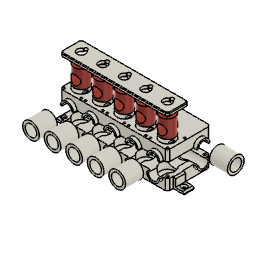
Luftstromverteilerkasten (Autodesk Fusion 360 design; units mm, degrees)
Autodesk Fusion 360 part; units mm, degrees
sketch "Skizze1" plane through (0, 0, 0) normal (0, 0, 1) x (1, 0, 0)
  line L0 (7, 22) -> (-8, 22)
  line L1 (-8, 22) -> (-8, -8)
  line L2 (-8, -8) -> (7, -8)
  line L3 (7, 22) -> (22, 22)
  line L4 (22, 22) -> (22, -8)
  line L5 (22, -8) -> (7, -8)
  line L6 (0.25, -0.3782) -> (0.25, -8)
  line L7 (0.25, -8) -> (7, -8)
  line L8 (13.75, -0.3782) -> (13.75, -8)
  line L9 (13.75, -8) -> (7, -8)
  circle A0 centre (7, 7) radius 10
  line L10 (0.25, -8) -> (0.25, 22)
  line L11 (13.75, -8) -> (13.75, 22)
  circle A1 centre (7, 7) radius 10.25
  dimension "d6" = 15
  dimension "d7" = 30
  dimension "d8" = 15
  dimension "d9" = 30
  dimension "d14" = 20
  dimension "d15" = 20.5
  constraint horizontal L0
  constraint vertical L1
  constraint horizontal L2
  constraint horizontal L3
  constraint vertical L4
  constraint horizontal L5
  constraint vertical L6
  constraint horizontal L7
  constraint vertical L8
  constraint horizontal L9
  constraint coincident A0 L6.start
  constraint coincident A0 L8.start
  constraint coincident L0 L10.end
  constraint perpendicular L0 L10
  constraint coincident L3 L11.end
  constraint perpendicular L3 L11
  constraint concentric A0 A1
  measures "d6" distance of L0.start L0.end
  measures "d7" distance of L0.start L2.end
  measures "d8" distance of L0.start L3.end
  measures "d9" distance of L0.start L2.end
  measures "d14" diameter of A0
  measures "d15" diameter of A1
  measures "d43" distance of L2.end
  measures "d44" distance of L2.end
extrude "Extrusion1" add sketch "Skizze1" along normal blind 30 contours L0 L3 L10 L11 A1 | L0 L1 L2 L6 L10 A1 | L3 L4 L5 L8 L11 A1 | L2 L5 L6 L7 L8 L9 L10 L11 A1 makes body 1
sketch "Skizze2" plane through (0, -8, 0) normal (0, -1, 0) x (1, 0, 0)
  line L0 (-8, 0) -> (22, 0)
  line L1 (22, 0) -> (22, 30)
  line L2 (22, 30) -> (-8, 30)
  line L3 (-8, 30) -> (-8, 0)
  line L4 (-8, 30) -> (22, 0)
  circle A0 centre (7, 15) radius 6.75
  dimension "d18" = 13.5
  constraint coincident L2.end L3.start
  constraint coincident L0.end L1.start
  constraint midpoint L4 A0.centre
  measures "d18" diameter of A0
extrude "Extrusion2" cut sketch "Skizze2" against normal blind 50 contours L4 A0 | L4 A0 bodies 1
extrude "Extrusion3" add sketch "Skizze1" along normal blind 5 contours A0 L10 L11 A1 | L6 A0 L10 A1 | L8 A0 L11 A1 | A0 L10 | A0 L10 L11 | L6 L8 A0 L10 L11 A1 | A0 L11 bodies 1
sketch "Skizze3" plane through (0, 0, 0) normal (0, 0, -1) x (1, 0, 0)
  line L0 (-8, -22) -> (22, -22)
  line L1 (22, -22) -> (22, 8)
  line L2 (22, 8) -> (-8, 8)
  line L3 (-8, 8) -> (-8, -22)
sketch "Skizze4" plane through (0, 0, 5) normal (0, 0, 1) x (-1, 0, 0)
  circle A0 centre (-7, -7) radius 10.25
  circle A1 centre (-7, -7) radius 2
  constraint concentric A0 A1
extrude "Extrusion4" add sketch "Skizze4" along normal blind 1 contours A1 bodies 1
sketch "Skizze5" plane through (0, 0, 5) normal (0, 0, 1) x (-1, 0, 0)
  circle A0 centre (-7, -7) radius 2
  circle A1 centre (-7, -7) radius 10.25
  circle A2 centre (-7, -7) radius 10
  circle A3 centre (-7, -7) radius 2.5
  dimension "d25" = 5
  constraint concentric A0 A2
  constraint concentric A2 A3
  measures "d25" diameter of A3
extrude "Extrusion5" add sketch "Skizze5" along normal blind 24.7 separate body contours A2 makes body 2
move_body "Verschieben1" bodies 2 to x (1, 0, 0) y (0, 1, 0) z (0, 0, 1) at (0, 0, 57)
sketch "Skizze6" plane through (0, 0, 86.7) normal (0, 0, 1) x (-1, 0, 0)
  circle A0 centre (-7, -7) radius 2.5
  circle A1 centre (-7, -7) radius 10
  circle A2 centre (-7, -7) radius 10
  constraint concentric A0 A2
extrude "Extrusion6" add sketch "Skizze6" against normal blind 23 contours A0 bodies 2
extrude "Extrusion7" add 1 faces at (8.044, 7.2271, 63.7) along direction (0, 0, -1) blind 0.7 on bodies 2 bodies 2
move_body "Verschieben2" bodies 2 to x (1, 0, 0) y (0, 1, 0) z (0, 0, 1) at (0, 0, -56.7)
extrude "Extrusion8" cut sketch "Skizze2" against normal blind 133 contours L4 A0 | L4 A0 bodies 2
sketch "Skizze7" plane through (0, 0, 30) normal (0, 0, 1) x (-1, 0, 0)
  circle A0 centre (-7, -7) radius 10
  circle A1 centre (-7, -7) radius 2.35
  dimension "d34" = 4.7
  constraint concentric A0 A1
  measures "d34" diameter of A1
extrude "Extrusion9" cut sketch "Skizze7" against normal blind 3.2 contours A1 bodies 2
sketch "Skizze8" plane through (0, 0, 30) normal (0, 0, 1) x (-1, 0, 0)
  circle A0 centre (-7, -7) radius 10.25
  line L0 (-22, -22) -> (8, -22)
  line L1 (8, -22) -> (8, 8)
  line L2 (8, 8) -> (-22, 8)
  line L3 (-22, 8) -> (-22, -22)
  line L4 (-22, -22) -> (8, 8)
  line L5 (8, -22) -> (-22, 8)
  line L6 (8, -22) -> (5, -22)
  line L7 (5, -22) -> (5, -19)
  line L8 (5, -19) -> (8, -19)
  line L9 (8, -19) -> (8, -22)
  line L10 (-22, -22) -> (-19, -22)
  line L11 (-19, -22) -> (-19, -19)
  line L12 (-19, -19) -> (-22, -19)
  line L13 (-22, -19) -> (-22, -22)
  line L14 (8, 8) -> (5, 8)
  line L15 (5, 8) -> (5, 5)
  line L16 (5, 5) -> (8, 5)
  line L17 (8, 5) -> (8, 8)
  line L18 (-22, 8) -> (-19, 8)
  line L19 (-19, 8) -> (-19, 5)
  line L20 (-19, 5) -> (-22, 5)
  line L21 (-22, 5) -> (-22, 8)
  circle A1 centre (5, 5) radius 1.5
  circle A2 centre (-19, 5) radius 1.5
  circle A3 centre (-19, -19) radius 1.5
  circle A4 centre (5, -19) radius 1.5
  dimension "d37" = 3
  dimension "d38" = 3
  dimension "d39" = 3
  dimension "d40" = 3
  dimension "d41" = 3
  dimension "d42" = 3
  dimension "d43" = 3
  dimension "d44" = 3
  constraint coincident L0.start L3.end
  constraint coincident L1.end L2.start
  constraint coincident L0.end L1.start
  constraint coincident L2.end L3.start
  constraint horizontal L6
  constraint vertical L7
  constraint horizontal L8
  constraint vertical L9
  constraint horizontal L10
  constraint vertical L11
  constraint horizontal L12
  constraint vertical L13
  constraint horizontal L14
  constraint vertical L15
  constraint horizontal L16
  constraint vertical L17
  constraint horizontal L18
  constraint vertical L19
  constraint horizontal L20
  constraint vertical L21
  constraint coincident L15.end L16.start
  constraint coincident L19.end L20.start
  constraint coincident L11.end L12.start
  constraint coincident L7.end L8.start
  measures "d37" distance of L0.end L6.end
  measures "d38" distance of L0.end L8.end
  measures "d39" distance of L0.start L10.end
  measures "d40" distance of L0.start L12.end
  measures "d41" distance of L1.end L14.end
  measures "d42" distance of L1.end L16.end
  measures "d43" distance of L2.end L18.end
  measures "d44" distance of L2.end L20.end
extrude "Extrusion10" cut sketch "Skizze8" against normal blind 2 contours L4 L15 A1 | L4 L16 A1 | L5 L8 A4 | L5 L7 A4 | L5 L20 A2 | L5 L19 A2 | L4 L15 A1 | L4 L16 A1 | L4 L11 A3 | L4 L12 A3 | L5 L8 A4 | L5 L7 A4 | L5 L20 A2 | L5 L19 A2 | L4 L11 A3 | L4 L12 A3 bodies 1
copy_body "Körper kopieren/einfügen1" bodies 2 1 makes body 3 makes body 4
move_body "Verschieben3" bodies 3 4 to x (1, 0, 0) y (0, 1, 0) z (0, 0, 1) at (30, 0, 0)
copy_body "Körper kopieren/einfügen2" bodies 3 4 1 2 makes body 5 makes body 6 makes body 7 makes body 8
move_body "Verschieben4" bodies 5 6 7 8 to x (1, 0, 0) y (0, 1, 0) z (0, 0, 1) at (60, 0, 0)
copy_body "Körper kopieren/einfügen3" bodies 5 6 makes body 9 makes body 10
move_body "Verschieben5" bodies 9 10 to x (1, 0, 0) y (0, 1, 0) z (0, 0, 1) at (30, 0, 0)
combine "Kombinieren1" operation add target body 1 tool bodies 4 7 6 10
sketch "Skizze9" plane through (0, 0, 0) normal (0, 1, 0) x (1, 0, 0)
sketch "Skizze10" plane through (0, 0, 30) normal (0, 0, 1) x (-1, 0, 0)
  circle A0 centre (-127, -7) radius 10.25
  circle A1 centre (-115, 5) radius 1.5
  circle A2 centre (-115, -19) radius 1.5
  circle A3 centre (-139, 5) radius 1.5
  circle A4 centre (-139, -19) radius 1.5
  circle A5 centre (-97, -7) radius 10.25
  circle A6 centre (-85, 5) radius 1.5
  circle A7 centre (-85, -19) radius 1.5
  circle A8 centre (-109, 5) radius 1.5
  circle A9 centre (-109, -19) radius 1.5
  circle A10 centre (-67, -7) radius 10.25
  circle A11 centre (-55, 5) radius 1.5
  circle A12 centre (-55, -19) radius 1.5
  circle A13 centre (-79, 5) radius 1.5
  circle A14 centre (-79, -19) radius 1.5
  circle A15 centre (-37, -7) radius 10.25
  circle A16 centre (-25, 5) radius 1.5
  circle A17 centre (-25, -19) radius 1.5
  circle A18 centre (-49, 5) radius 1.5
  circle A19 centre (-49, -19) radius 1.5
  circle A20 centre (-19, -19) radius 1.5
  circle A21 centre (-19, 5) radius 1.5
  circle A22 centre (5, -19) radius 1.5
  circle A23 centre (5, 5) radius 1.5
  circle A24 centre (-7, -7) radius 10.25
  line L0 (-142, -22) -> (8, -22)
  line L1 (8, -22) -> (8, 8)
  line L2 (8, 8) -> (-142, 8)
  line L3 (-142, 8) -> (-142, -22)
  line L4 (8, -22) -> (-142, -22)
  line L5 (-142, -22) -> (-142, 8)
  line L6 (-142, 8) -> (8, 8)
  line L7 (8, 8) -> (8, -22)
  circle A25 centre (-7, -7) radius 5.9
  circle A26 centre (-37, -7) radius 5.9
  circle A27 centre (-67, -7) radius 5.9
  circle A28 centre (-97, -7) radius 5.9
  circle A29 centre (-127, -7) radius 5.9
  line L8 (-7, -7) -> (-7, -15.8)
  line L9 (-37, -7) -> (-37, -15.8)
  line L10 (-67, -7) -> (-67, -15.8)
  line L11 (-97, -7) -> (-97, -15.8)
  line L12 (-127, -7) -> (-127, -15.8)
  circle A30 centre (-7, -13.3) radius 2.5
  circle A31 centre (-37, -13.3) radius 2.5
  circle A32 centre (-67, -13.3) radius 2.5
  circle A33 centre (-97, -13.3) radius 2.5
  circle A34 centre (-127, -13.3) radius 2.5
  line L13 (-7, -13.3) -> (-4.5, -13.3)
  line L14 (-4.5, -13.3) -> (-4.5, -12.3442)
  line L15 (-7, -13.3) -> (-9.5, -13.3)
  line L16 (-9.5, -13.3) -> (-9.5, -12.3442)
  line L17 (-37, -13.3) -> (-34.5, -13.3)
  line L18 (-34.5, -13.3) -> (-34.5, -12.3442)
  line L19 (-37, -13.3) -> (-39.5, -13.3)
  line L20 (-39.5, -13.3) -> (-39.5, -12.3442)
  line L21 (-67, -13.3) -> (-64.5, -13.3)
  line L22 (-64.5, -13.3) -> (-64.5, -12.3442)
  line L23 (-67, -13.3) -> (-69.5, -13.3)
  line L24 (-69.5, -13.3) -> (-69.5, -12.3442)
  line L25 (-97, -13.3) -> (-94.5, -13.3)
  line L26 (-94.5, -13.3) -> (-94.5, -12.3442)
  line L27 (-97, -13.3) -> (-99.5, -13.3)
  line L28 (-99.5, -13.3) -> (-99.5, -12.3442)
  line L29 (-127, -13.3) -> (-124.5, -13.3)
  line L30 (-124.5, -13.3) -> (-124.5, -12.3442)
  line L31 (-127, -13.3) -> (-129.5, -13.3)
  line L32 (-129.5, -13.3) -> (-129.5, -12.3442)
  circle A35 centre (5, -19) radius 1.3
  circle A36 centre (-19, -19) radius 1.3
  circle A37 centre (-25, -19) radius 1.3
  circle A38 centre (-49, -19) radius 1.3
  circle A39 centre (-55, -19) radius 1.3
  circle A40 centre (-79, -19) radius 1.3
  circle A41 centre (-85, -19) radius 1.3
  circle A42 centre (-109, -19) radius 1.3
  circle A43 centre (-115, -19) radius 1.3
  circle A44 centre (-139, -19) radius 1.3
  circle A45 centre (-139, 5) radius 1.3
  circle A46 centre (-115, 5) radius 1.3
  circle A47 centre (-109, 5) radius 1.3
  circle A48 centre (-85, 5) radius 1.3
  circle A49 centre (-79, 5) radius 1.3
  circle A50 centre (-55, 5) radius 1.3
  circle A51 centre (-49, 5) radius 1.3
  circle A52 centre (-25, 5) radius 1.3
  circle A53 centre (-19, 5) radius 1.3
  circle A54 centre (5, 5) radius 1.3
  dimension "d47" = 11.8
  dimension "d48" = 11.8
  dimension "d49" = 11.8
  dimension "d50" = 11.8
  dimension "d51" = 11.8
  dimension "d52" = 8.8
  dimension "d53" = 8.8
  dimension "d54" = 8.8
  dimension "d55" = 8.8
  dimension "d56" = 8.8
  dimension "d57" = 5
  dimension "d58" = 5
  dimension "d59" = 5
  dimension "d60" = 5
  dimension "d61" = 5
  dimension "d62" = 2.6
  dimension "d63" = 2.6
  dimension "d64" = 2.6
  dimension "d65" = 2.6
  dimension "d66" = 2.6
  dimension "d67" = 2.6
  dimension "d68" = 2.6
  dimension "d69" = 2.6
  dimension "d70" = 2.6
  dimension "d71" = 2.6
  dimension "d72" = 2.6
  dimension "d73" = 2.6
  dimension "d74" = 2.6
  dimension "d75" = 2.6
  dimension "d76" = 2.6
  dimension "d77" = 2.6
  dimension "d78" = 2.6
  dimension "d79" = 2.6
  dimension "d80" = 2.6
  dimension "d81" = 2.6
  constraint horizontal L4
  constraint vertical L5
  constraint horizontal L6
  constraint vertical L7
  constraint coincident L2.end L3.start
  constraint coincident L0.end L1.start
  constraint concentric A24 A25
  constraint concentric A15 A26
  constraint concentric A10 A27
  constraint concentric A5 A28
  constraint concentric A0 A29
  constraint coincident A24.centre A25.centre
  constraint perpendicular L4 L8
  constraint coincident A15.centre A26.centre
  constraint vertical L9
  constraint coincident A10.centre A27.centre
  constraint vertical L10
  constraint coincident A5.centre A28.centre
  constraint perpendicular L6 L11
  constraint coincident A0.centre A29.centre
  constraint vertical L12
  constraint coincident L8.end A30
  constraint coincident L9.end A31
  constraint coincident L10.end A32
  constraint coincident L11.end A33
  constraint coincident L12.end A34
  constraint coincident A30.centre L13.start
  constraint coincident A30 L13.end
  constraint perpendicular L8 L13
  constraint coincident A25 L14.end
  constraint tangent A30 L14
  constraint coincident A30 L15.end
  constraint perpendicular L8 L15
  constraint coincident A25 L16.end
  constraint perpendicular L15 L16
  constraint coincident A31.centre L17.start
  constraint coincident A31 L17.end
  constraint perpendicular L9 L17
  constraint coincident A26 L18.end
  constraint perpendicular L17 L18
  constraint coincident A31 L19.end
  constraint perpendicular L9 L19
  constraint coincident A26 L20.end
  constraint perpendicular L19 L20
  constraint coincident A32.centre L21.start
  constraint coincident A32 L21.end
  constraint perpendicular L10 L21
  constraint coincident A27 L22.end
  constraint perpendicular L21 L22
  constraint coincident A32 L23.end
  constraint perpendicular L10 L23
  constraint perpendicular L23 L24
  constraint coincident A33.centre L25.start
  constraint coincident A33 L25.end
  constraint perpendicular L11 L25
  constraint coincident A28 L26.end
  constraint perpendicular L25 L26
  constraint coincident A33 L27.end
  constraint perpendicular L11 L27
  constraint coincident A28 L28.end
  constraint perpendicular L27 L28
  constraint coincident A34.centre L29.start
  constraint coincident A34 L29.end
  constraint perpendicular L12 L29
  constraint coincident A29 L30.end
  constraint perpendicular L29 L30
  constraint coincident A34 L31.end
  constraint perpendicular L12 L31
  constraint coincident A29 L32.end
  constraint perpendicular L29 L32
  constraint concentric A22 A35
  constraint concentric A20 A36
  constraint concentric A17 A37
  constraint concentric A19 A38
  constraint concentric A12 A39
  constraint concentric A14 A40
  constraint concentric A7 A41
  constraint concentric A9 A42
  constraint concentric A2 A43
  constraint concentric A4 A44
  constraint concentric A3 A45
  constraint concentric A1 A46
  constraint concentric A8 A47
  constraint concentric A6 A48
  constraint concentric A13 A49
  constraint concentric A11 A50
  constraint concentric A18 A51
  constraint concentric A16 A52
  constraint concentric A21 A53
  constraint concentric A23 A54
  measures "d47" diameter of A25
  measures "d48" diameter of A26
  measures "d49" diameter of A27
  measures "d50" diameter of A28
  measures "d51" diameter of A29
  measures "d52" distance of A24.centre L8.end
  measures "d53" distance of A15.centre L9.end
  measures "d54" distance of A10.centre L10.end
  measures "d55" distance of A5.centre L11.end
  measures "d56" distance of A0.centre L12.end
  measures "d57" diameter of A30
  measures "d58" diameter of A31
  measures "d59" diameter of A32
  measures "d60" diameter of A33
  measures "d61" diameter of A34
  measures "d62" diameter of A35
  measures "d63" diameter of A36
  measures "d64" diameter of A37
  measures "d65" diameter of A38
  measures "d66" diameter of A39
  measures "d67" diameter of A40
  measures "d68" diameter of A41
  measures "d69" diameter of A42
  measures "d70" diameter of A43
  measures "d71" diameter of A44
  measures "d72" diameter of A45
  measures "d73" diameter of A46
  measures "d74" diameter of A47
  measures "d75" diameter of A48
  measures "d76" diameter of A49
  measures "d77" diameter of A50
  measures "d78" diameter of A51
  measures "d79" diameter of A52
  measures "d80" diameter of A53
  measures "d81" diameter of A54
move_body "Verschieben6" bodies 1 5 8 to x (1, 0, 0) y (0, 1, 0) z (0, 0, 1) at (0, 0, -15)
move_body "Verschieben7" bodies 2 3 9 to x (1, 0, 0) y (0, 1, 0) z (0, 0, 1) at (0, 0, -15)
extrude "Extrusion11" add sketch "Skizze10" along normal blind 2 separate body contours A0 | A1 | A2 | A3 | A4 | A5 | A6 | A7 | A8 | A9 | A10 | A11 | A12 | A13 | A14 | A15 | A16 | A17 | A18 | A19 | A20 | A21 | A22 | A23 | A24 | L0 L1 L2 L3 L4 L5 L6 L7 | A35 | A36 | A37 | A38 | A39 | A40 | A41 | A42 | A43 | A44 | A45 | A46 | A47 | A48 | A49 | A50 | A51 | A52 | A53 | A54 makes body 11
extrude "Extrusion12" add sketch "Skizze10" against normal blind 2 contours A35 | A36 | A37 | A38 | A39 | A40 | A41 | A42 | A43 | A44 | A45 | A46 | A47 | A48 | A49 | A50 | A51 | A52 | A53 | A54 bodies 11
extrude "Extrusion13" cut 20 faces at (-5.1917, -5.3235, 28) (-5.3026, 18.2291, 28) (18.5623, -4.812, 28) (19.3724, 18.5636, 28) (25.3724, 18.5636, 28) (24.5623, -4.812, 28) (48.1382, -5.0646, 28) (49.0464, 18.6612, 28) (55.0464, 18.6612, 28) (54.0847, -5.0281, 28) (84.642, -5.3733, 28) (78.642, -5.3733, 28) (78.642, 18.6267, 28) (84.642, 18.6267, 28) (108.642, -5.3733, 28) (114.642, -5.3733, 28) (108.642, 18.6267, 28) (114.642, 18.6267, 28) (138.6823, -5.4239, 28) (138.6096, 19.188, 28) along direction (0, 0, 1) blind 0.2 on bodies 11 bodies 11
move_body "Verschieben8" bodies 11 to x (1, 0, 0) y (0, 1, 0) z (0, 0, 1) at (0, 0, 30)
move_body "Verschieben9" bodies 2 3 1 5 9 8 to x (1, 0, 0) y (0, 1, 0) z (0, 0, 1) at (-67, 0, 15)
move_body "Verschieben10" bodies 11 to x (1, 0, 0) y (0, 1, 0) z (0, 0, 1) at (-67, 0, -30)
sketch "Skizze11" plane through (0, 0, 0) normal (0, 0, 1) x (1, 0, 0)
  line L0 (-107.8085, 14.3255) -> (-82.0961, 14.3255)
  line L1 (-82.0961, 14.3255) -> (-82.0961, -4.2242)
  line L2 (-82.0961, -4.2242) -> (-107.8085, -4.2242)
  line L3 (-107.8085, -4.2242) -> (-107.8085, 14.3255)
  constraint horizontal L0
  constraint vertical L1
  constraint horizontal L2
  constraint vertical L3
extrude "Extrusion14" add sketch "Skizze11" along normal blind 15 separate body makes body 12
split "Teilen1" by plane through (0, 0, 15) normal (0, 0, 1) bodies 1 makes body 13 at (14.2202, 12.5653, 30)
extrude "Extrusion15" cut 1 faces at (-99.2377, 1.959, 15) along direction (0, 0, -1) blind 35 on bodies 12 bodies 12
sketch "Skizze12" plane through (0, -8, 0) normal (0, -1, 0) x (1, 0, 0)
  line L0 (66.75, 15) -> (75, 15)
  line L1 (75, 15) -> (75, 30)
  line L2 (75, 30) -> (-75, 30)
  line L3 (-75, 30) -> (-75, 15)
  line L4 (-75, 15) -> (-66.75, 15)
  arc A0 (-53.25, 15) -> (-66.75, 15) centre (-60, 15) ccw
  line L5 (-53.25, 15) -> (-36.75, 15)
  arc A1 (-23.25, 15) -> (-36.75, 15) centre (-30, 15) ccw
  line L6 (-23.25, 15) -> (-6.75, 15)
  arc A2 (6.75, 15) -> (-6.75, 15) centre (0, 15) ccw
  line L7 (6.75, 15) -> (23.25, 15)
  arc A3 (36.75, 15) -> (23.25, 15) centre (30, 15) ccw
  line L8 (36.75, 15) -> (53.25, 15)
  arc A4 (66.75, 15) -> (53.25, 15) centre (60, 15) ccw
  circle A5 centre (-60, 15) radius 9
  circle A6 centre (-30, 15) radius 9
  circle A7 centre (0, 15) radius 9
  circle A8 centre (30, 15) radius 9
  circle A9 centre (60, 15) radius 9
  circle A10 centre (-60, 15) radius 6.75
  circle A11 centre (-30, 15) radius 6.75
  circle A12 centre (0, 15) radius 6.75
  circle A13 centre (30, 15) radius 6.75
  circle A14 centre (60, 15) radius 6.75
  dimension "d92" = 18
  dimension "d93" = 18
  dimension "d94" = 18
  dimension "d95" = 18
  dimension "d96" = 18
  constraint concentric A0 A5
  constraint concentric A1 A6
  constraint concentric A2 A7
  constraint concentric A3 A8
  constraint concentric A4 A9
  constraint concentric A5 A10
  constraint concentric A6 A11
  constraint concentric A7 A12
  constraint concentric A8 A13
  constraint concentric A9 A14
  measures "d92" diameter of A5
  measures "d93" diameter of A6
  measures "d94" diameter of A7
  measures "d95" diameter of A8
  measures "d96" diameter of A9
extrude "Extrusion16" add sketch "Skizze12" along normal blind 5 contours L0 L8 A4 A9 A14 | L7 A3 L8 A8 A13 | L6 A2 L7 A7 A12 | L4 A0 L5 A5 A10 | L5 A1 L6 A6 A11 bodies 12 1 13
extrude "Extrusion17" add sketch "Skizze12" along normal blind 5 contours L0 L8 A9 A14 | L7 L8 A8 A13 | L6 L7 A7 A12 | L4 L5 A5 A10 | L5 L6 A6 A11 bodies 12
sketch "Skizze13" plane through (75, 0, 0) normal (1, 0, 0) x (0, 1, 0)
  line L0 (-8, 30) -> (-8, 0)
  line L1 (-8, 0) -> (22, 0)
  line L2 (22, 0) -> (22, 30)
  line L3 (22, 30) -> (-8, 30)
  line L4 (7, 0) -> (7, 15)
  line L5 (7, 15) -> (0, 15)
  line L6 (0, 15) -> (0, 0)
  line L7 (0, 0) -> (7, 0)
  line L8 (7, 0) -> (7, 15)
  line L9 (7, 15) -> (14, 15)
  line L10 (14, 15) -> (14, 0)
  line L11 (14, 0) -> (7, 0)
  line L12 (7, 0) -> (7, 15)
  line L13 (0, 0) -> (14, 0)
  line L14 (14, 0) -> (14, 3)
  line L15 (14, 3) -> (0, 3)
  line L16 (0, 3) -> (0, 0)
  constraint midpoint L1 L4.start
  constraint perpendicular L1 L4
  constraint horizontal L5
  constraint vertical L6
  constraint horizontal L7
  constraint vertical L8
  constraint coincident L6.end L7.start
  constraint horizontal L9
  constraint vertical L10
  constraint horizontal L11
  constraint vertical L12
  constraint coincident L1 L10.end
  constraint horizontal L13
  constraint vertical L14
  constraint horizontal L15
  constraint vertical L16
  constraint coincident L10 L14.end
extrude "Extrusion18" add sketch "Skizze13" along normal blind 3 contours L4 L5 L6 L8 L12 L15 | L4 L8 L9 L10 L12 L15 bodies 12
extrude "Extrusion19" add sketch "Skizze13" along normal blind 15 contours L1 L4 L6 L7 L8 L12 L13 L15 L16 | L1 L4 L8 L10 L11 L12 L13 L14 L15 bodies 12
chamfer "Fase1" distance 2 angle 45 2 edges at (78, 7, 15) (90, 7, 3) on bodies 12
sketch "Skizze14" plane through (0, 0, 3) normal (0, 0, 1) x (-1, 0, 0)
  line L0 (-88, 0) -> (-88, -14)
  line L1 (-88, -14) -> (-78, -14)
  line L2 (-78, -14) -> (-78, 0)
  line L3 (-78, 0) -> (-88, 0)
  circle A0 centre (-83, -7) radius 2
extrude "Extrusion20" cut sketch "Skizze14" against normal blind 4 contours A0 bodies 12
chamfer "Fase2" distance 2 angle 45 1 edges at (84.8647, 6.2768, 3) on bodies 12
sketch "Skizze15" plane through (-75, 0, 0) normal (-1, 0, 0) x (0, -1, 0)
  line L0 (-22, 30) -> (-22, 0)
  line L1 (-22, 0) -> (8, 0)
  line L2 (8, 0) -> (8, 30)
  line L3 (8, 30) -> (-22, 30)
  line L4 (-7, 0) -> (-7, 15)
  line L5 (-7, 15) -> (0, 15)
  line L6 (0, 15) -> (-7, 15)
  line L7 (-7, 15) -> (-14, 15)
  line L8 (-14, 15) -> (-14, 0)
  line L9 (0, 15) -> (0, 0)
  line L10 (-14, 0) -> (-14, 3)
  line L11 (-14, 3) -> (0, 3)
  line L12 (0, 3) -> (0, 0)
  line L13 (0, 0) -> (-14, 0)
  line L14 (-14, 0) -> (-14, 3)
  dimension "d109" = 15
  dimension "d110" = 7
  dimension "d111" = 7
  dimension "d112" = 7
  constraint midpoint L1 L4.start
  constraint perpendicular L1 L4
  constraint perpendicular L4 L5
  constraint perpendicular L4 L6
  constraint perpendicular L4 L7
  constraint coincident L1 L8.end
  constraint perpendicular L1 L8
  constraint coincident L9.end L12.end
  constraint coincident L8 L10.end
  constraint horizontal L11
  constraint vertical L12
  constraint horizontal L13
  constraint vertical L14
  measures "d109" distance of L4.start L4.end
  measures "d110" distance of L4.end L5.end
  measures "d111" distance of L5.end L4.end
  measures "d112" distance of L4.end L7.end
extrude "Extrusion21" add sketch "Skizze15" along normal blind 3 contours L4 L7 L8 L11 | L4 L5 L6 L9 L11 bodies 12
extrude "Extrusion22" add sketch "Skizze15" along normal blind 15 contours L1 L4 L8 L10 L11 L13 L14 | L1 L4 L9 L11 L12 L13 bodies 12
sketch "Skizze16" plane through (0, 0, 3) normal (0, 0, 1) x (-1, 0, 0)
  line L0 (78, 0) -> (78, -14)
  line L1 (78, -14) -> (90, -14)
  line L2 (90, -14) -> (90, 0)
  line L3 (90, 0) -> (78, 0)
chamfer "Fase3" distance 2 angle 45 2 edges at (-78, 7, 15) (-90, 7, 3) on bodies 12
sketch "Skizze17" plane through (0, 0, 3) normal (0, 0, 1) x (-1, 0, 0)
  circle A0 centre (83, -7) radius 2
extrude "Extrusion23" cut sketch "Skizze17" against normal blind 10 bodies 12
chamfer "Fase4" distance 2 angle 45 1 edges at (-81.1353, 6.2768, 3) on bodies 12
chamfer "Fase5" distance 3 angle 45 8 edges at (-75, -8, 31) (75, -8, 31) (75, 22, 31) (-75, 22, 31) (-75, -8, 15) (75, -8, 15) (75, 22, 15) (-75, 22, 15) on bodies 11 12
chamfer "Fase6" distance 1 angle 45 8 edges at (0, 22, 32) (75, 7, 32) (73.5, 20.5, 32) (73.5, -6.5, 32) (0, -8, 32) (-73.5, -6.5, 32) (-75, 7, 32) (-73.5, 20.5, 32) on bodies 11
sketch "Skizze18" plane through (0, 0, 0) normal (0, 0, 1) x (1, 0, 0)
sketch "Skizze19" plane through (0, 0, 0) normal (0, 0, 1) x (1, 0, 0)
  line L0 (75, 19) -> (-75, 19)
  line L1 (-75, 19) -> (-75, 22)
  line L2 (-75, 22) -> (75, 22)
  line L3 (75, 22) -> (75, 19)
  line L4 (-75, 22) -> (75, 22)
  line L5 (75, 22) -> (75, 52)
  line L6 (75, 52) -> (-75, 52)
  line L7 (-75, 52) -> (-75, 22)
  line L8 (72, 22) -> (75, 19)
  line L9 (-72, 22) -> (-75, 19)
  dimension "d123" = 30
  constraint horizontal L0
  constraint vertical L1
  constraint horizontal L2
  constraint vertical L3
  constraint horizontal L4
  constraint vertical L5
  constraint horizontal L6
  constraint vertical L7
  constraint coincident L4 L8.start
  constraint coincident L2 L9.start
  constraint perpendicular L8 L9
  measures "d123" distance of L1.end L6.end
move_body "Verschieben11" bodies 11 to x (1, 0, 0) y (0, 1, 0) z (0, 0, 1) at (0, 0, 15)
extrude "Extrusion24" add sketch "Skizze19" along normal blind 30 contours L2 L3 L4 L8 | L1 L2 L4 L9 | L2 L4 L5 L6 L7 bodies 12
sketch "Skizze20" plane through (75, 0, 0) normal (1, 0, 0) x (0, 1, 0)
  line L0 (52, 30) -> (-5, 30)
  line L1 (-5, 30) -> (-5, 0)
  line L2 (-5, 0) -> (0, 0)
  line L3 (0, 0) -> (0, 15)
  line L4 (0, 15) -> (14, 15)
  line L5 (14, 15) -> (14, 0)
  line L6 (14, 0) -> (52, 0)
  line L7 (52, 0) -> (52, 30)
  line L8 (52, 30) -> (-8, 30)
  line L9 (-8, 30) -> (-8, 0)
  line L10 (-8, 0) -> (52, 0)
  line L11 (52, 0) -> (52, 30)
  line L12 (52, 30) -> (22, 30)
  line L13 (22, 30) -> (22, 0)
  line L14 (22, 0) -> (52, 0)
  line L15 (52, 0) -> (52, 30)
  line L16 (22, 30) -> (52, 0)
  circle A0 centre (37, 15) radius 6.75
  dimension "d126" = 60
  dimension "d127" = 30
  dimension "d128" = 13.5
  constraint horizontal L8
  constraint vertical L9
  constraint horizontal L10
  constraint vertical L11
  constraint coincident L0.start L7.end
  constraint horizontal L12
  constraint vertical L13
  constraint horizontal L14
  constraint vertical L15
  constraint coincident L6.end L7.start
  constraint midpoint L16 A0.centre
  measures "d126" distance of L0.start L8.end
  measures "d127" distance of L0.start L12.end
  measures "d128" diameter of A0
extrude "Extrusion25" cut sketch "Skizze20" against normal blind 195 contours L16 A0 | L16 A0 bodies 12
sketch "Skizze21" plane through (0, -13, 0) normal (0, -1, 0) x (1, 0, 0)
  circle A0 centre (-60, 15) radius 9
  circle A1 centre (-60, 15) radius 6.75
  circle A2 centre (-60, 15) radius 6.75
  circle A3 centre (-30, 15) radius 6.75
  circle A4 centre (0, 15) radius 6.75
  circle A5 centre (30, 15) radius 6.75
  circle A6 centre (60, 15) radius 6.75
  dimension "d131" = 13.5
  dimension "d132" = 13.5
  dimension "d133" = 13.5
  dimension "d134" = 13.5
  constraint concentric A0 A2
  measures "d131" diameter of A3
  measures "d132" diameter of A4
  measures "d133" diameter of A5
  measures "d134" diameter of A6
extrude "Extrusion26" cut sketch "Skizze21" against normal blind 50 contours A1 A2 | A3 | A4 | A5 | A6 bodies 12
sketch "Skizze22" plane through (-75, 0, 0) normal (-1, 0, 0) x (0, -1, 0)
  circle A0 centre (-37, 15) radius 6.75
  line L0 (-52, 0) -> (-14, 0)
  line L1 (-14, 0) -> (-14, 15)
  line L2 (-14, 15) -> (0, 15)
  line L3 (0, 15) -> (0, 3)
  line L4 (0, 3) -> (0, 0)
  line L5 (0, 0) -> (5, 0)
  line L6 (5, 0) -> (5, 30)
  line L7 (5, 30) -> (-52, 30)
  line L8 (-52, 30) -> (-52, 0)
  circle A1 centre (-37, 15) radius 6.75
  constraint concentric A0 A1
extrude "Extrusion27" add sketch "Skizze22" against normal blind 3 contours A0 A1 bodies 12
fillet "Abrundung1" radius 3 10 edges at (-66.75, 30.25, 15) (-53.25, 30.25, 15) (-36.75, 30.25, 15) (-23.25, 30.25, 15) (-6.75, 30.25, 15) (6.75, 30.25, 15) (23.25, 30.25, 15) (36.75, 30.25, 15) (53.25, 30.25, 15) (66.75, 30.25, 15) on bodies 12
sketch "Skizze23" plane through (75, 0, 0) normal (1, 0, 0) x (0, 1, 0)
  circle A0 centre (37, 15) radius 6.75
  line L0 (52, 30) -> (-5, 30)
  line L1 (-5, 30) -> (-5, 0)
  line L2 (-5, 0) -> (0, 0)
  line L3 (0, 0) -> (0, 15)
  line L4 (0, 15) -> (14, 15)
  line L5 (14, 15) -> (14, 0)
  line L6 (14, 0) -> (52, 0)
  line L7 (52, 0) -> (52, 30)
  circle A1 centre (37, 15) radius 9
  dimension "d141" = 18
  constraint concentric A0 A1
  measures "d141" diameter of A1
extrude "Extrusion28" add sketch "Skizze23" along normal blind 5 contours A1 bodies 12
chamfer "Fase7" distance 3 angle 45 2 edges at (75, 52, 15) (-75, 52, 15) on bodies 12
split "Teilen2" by plane through (75, 7, 15) normal (0, 0, 1) bodies 12 makes body 14 at (-3.9477, 41.4973, 30)
move_body "Verschieben12" bodies 11 to x (1, 0, 0) y (0, 1, 0) z (0, 0, 1) at (0, -110, 0)
move_body "Verschieben13" bodies 14 to x (1, 0, 0) y (0, 1, 0) z (0, 0, 1) at (0, 100, 0)
move_body "Verschieben14" bodies 2 3 8 5 9 to x (1, 0, 0) y (0, 1, 0) z (0, 0, 1) at (0, -50, 0)
sketch "Skizze24" plane through (0, 0, 15) normal (0, 0, 1) x (-1, 0, 0)
  line L0 (-76, 0) -> (-76, -14)
  line L1 (-76, -14) -> (-75, -14)
  line L2 (-75, -14) -> (-75, -28)
  line L3 (-75, -28) -> (-80, -28)
  line L4 (-80, -28) -> (-80, -30.25)
  line L5 (-80, -30.25) -> (-69.75, -30.25)
  spline S0 degree 3 poles (-69.75, -30.25) (-69.5486, -30.25) (-69.3476, -30.2297) (-68.9529, -30.1492) (-68.7601, -30.0891) (-68.2153, -29.8572) (-67.8892, -29.6354) (-67.3404, -29.0793) (-67.1229, -28.7503) (-66.8263, -28.0276) (-66.75, -27.6406) (-66.75, -27.25) knots -0.472444 -0.472444 -0.472444 -0.472444 -0.412012 -0.412012 -0.35158 -0.35158 -0.234387 -0.234387 -0.117193 -0.117193 0 0 0 0
  line L6 (-66.75, -27.25) -> (-66.75, -14.7136)
  arc A0 (-66.75, 0.7136) -> (-66.75, -14.7136) centre (-60, -7) ccw
  line L7 (-66.75, 0.7136) -> (-66.75, 13)
  line L8 (-66.75, 13) -> (-69, 13)
  line L9 (-69, 13) -> (-69, 8)
  line L10 (-69, 8) -> (-72, 8)
  line L11 (-72, 8) -> (-75, 5)
  line L12 (-75, 5) -> (-75, 0)
  line L13 (-75, 0) -> (-76, 0)
  circle A1 centre (-71, 4) radius 2
  circle A2 centre (-71, -48) radius 2
  circle A3 centre (71, 4) radius 2
  circle A4 centre (71, -48) radius 2
extrude "Extrusion29" cut sketch "Skizze24" against normal blind 2 contours A1 | A2 | A3 | A4 bodies 12
sketch "Skizze25" plane through (0, 0, 15) normal (0, 0, -1) x (1, 0, 0)
  line L0 (-75, -95) -> (-75, -149)
  line L1 (-75, -149) -> (-72, -152)
  line L2 (-72, -152) -> (72, -152)
  line L3 (72, -152) -> (75, -149)
  line L4 (75, -149) -> (75, -146)
  line L5 (75, -146) -> (80, -146)
  line L6 (80, -146) -> (80, -143.75)
  line L7 (80, -143.75) -> (-72, -143.75)
  line L8 (-72, -143.75) -> (-72, -130.25)
  line L9 (-72, -130.25) -> (-69.75, -130.25)
  spline S0 degree 3 poles (-66.75, -127.25) (-66.75, -127.4514) (-66.7703, -127.6524) (-66.8508, -128.0471) (-66.9109, -128.2399) (-67.1428, -128.7847) (-67.3646, -129.1108) (-67.9207, -129.6596) (-68.2497, -129.8771) (-68.9724, -130.1737) (-69.3594, -130.25) (-69.75, -130.25) knots -0.472444 -0.472444 -0.472444 -0.472444 -0.412012 -0.412012 -0.35158 -0.35158 -0.234387 -0.234387 -0.117193 -0.117193 0 0 0 0
  line L10 (-66.75, -127.25) -> (-66.75, -114.7136)
  arc A0 (-66.75, -99.2864) -> (-66.75, -114.7136) centre (-60, -107) ccw
  line L11 (-66.75, -99.2864) -> (-66.75, -87)
  line L12 (-66.75, -87) -> (-69, -87)
  line L13 (-69, -87) -> (-69, -92)
  line L14 (-69, -92) -> (-72, -92)
  line L15 (-72, -92) -> (-75, -95)
  circle A1 centre (71, -148) radius 1.9
  circle A2 centre (-71, -148) radius 1.9
  circle A3 centre (-71, -96) radius 1.9
  circle A4 centre (71, -96) radius 1.9
  dimension "d147" = 3.8
  dimension "d148" = 3.8
  dimension "d149" = 3.8
  dimension "d150" = 3.8
  measures "d147" diameter of A1
  measures "d148" diameter of A2
  measures "d149" diameter of A3
  measures "d150" diameter of A4
extrude "Extrusion30" add sketch "Skizze25" along normal blind 1.8 contours A1 | A2 | A3 | A4 bodies 14
extrude "Extrusion31" add 20 faces at (-71.6978, -115.8699, 43.2) (-47.5859, -115.1277, 43.2) (-41.5859, -115.1277, 43.2) (-17.6545, -115.3849, 43.2) (-11.6545, -115.3849, 43.2) (11.6144, -115.1234, 43.2) (17.6144, -115.1234, 43.2) (41.642, -114.6267, 43.2) (47.642, -114.6267, 43.2) (72.4141, -115.1277, 43.2) (72.4141, -91.1277, 43.2) (48.4141, -91.1277, 43.2) (42.4141, -91.1277, 43.2) (17.6096, -91.188, 43.2) (11.6096, -91.188, 43.2) (-12.9202, -90.9635, 43.2) (-18.9202, -90.9635, 43.2) (-41.7298, -90.2852, 43.2) (-47.7298, -90.2852, 43.2) (-72.4333, -90.7445, 43.2) along direction (0, 0, -1) blind 2 on bodies 11 bodies 11
extrude "Extrusion32" add 1 faces at (44.1243, -98.983, 45) along direction (0, 0, -1) blind 2 on bodies 11 bodies 11
sketch "Skizze26" plane through (0, 0, 47) normal (0, 0, 1) x (-1, 0, 0)
  line L0 (-27.5, 97.6558) -> (-27.5, 96.7)
  arc A0 (-32.5, 96.7) -> (-27.5, 96.7) centre (-30, 96.7) ccw
  line L1 (-32.5, 96.7) -> (-32.5, 97.6558)
  arc A1 (-27.5, 97.6558) -> (-32.5, 97.6558) centre (-30, 103) ccw
  line L2 (-57.5, 97.6558) -> (-57.5, 96.7)
  arc A2 (-62.5, 96.7) -> (-57.5, 96.7) centre (-60, 96.7) ccw
  line L3 (-62.5, 96.7) -> (-62.5, 97.6558)
  arc A3 (-57.5, 97.6558) -> (-62.5, 97.6558) centre (-60, 103) ccw
  line L4 (32.5, 97.6558) -> (32.5, 96.7)
  arc A4 (27.5, 96.7) -> (32.5, 96.7) centre (30, 96.7) ccw
  line L5 (27.5, 96.7) -> (27.5, 97.6558)
  arc A5 (32.5, 97.6558) -> (27.5, 97.6558) centre (30, 103) ccw
  line L6 (2.5, 97.6558) -> (2.5, 96.7)
  arc A6 (-2.5, 96.7) -> (2.5, 96.7) centre (0, 96.7) ccw
  line L7 (-2.5, 96.7) -> (-2.5, 97.6558)
  arc A7 (2.5, 97.6558) -> (-2.5, 97.6558) centre (0, 103) ccw
  line L8 (62.5, 97.6558) -> (62.5, 96.7)
  arc A8 (57.5, 96.7) -> (62.5, 96.7) centre (60, 96.7) ccw
  line L9 (57.5, 96.7) -> (57.5, 97.6558)
  arc A9 (62.5, 97.6558) -> (57.5, 97.6558) centre (60, 103) ccw
  line L10 (71.5858, 117) -> (-71.5858, 117)
  line L11 (-71.5858, 117) -> (-74, 114.5858)
  line L12 (-74, 114.5858) -> (-74, 91.4142)
  line L13 (-74, 91.4142) -> (-71.5858, 89)
  line L14 (-71.5858, 89) -> (71.5858, 89)
  line L15 (71.5858, 89) -> (74, 91.4142)
  line L16 (74, 91.4142) -> (74, 114.5858)
  line L17 (74, 114.5858) -> (71.5858, 117)
  line L18 (60, 103) -> (-60, 103)
  line L19 (60, 103) -> (30, 103)
  line L20 (30, 103) -> (0, 103)
  line L21 (0, 103) -> (-30, 103)
  line L22 (-30, 103) -> (-60, 103)
  line L23 (30, 103) -> (60, 103)
  line L24 (45, 103) -> (45, 89)
  line L25 (45, 103) -> (45, 117)
  line L26 (15, 103) -> (15, 89)
  line L27 (15, 103) -> (15, 117)
  line L28 (-15, 103) -> (-15, 89)
  line L29 (-15, 103) -> (-15, 117)
  line L30 (-45, 103) -> (-45, 89)
  line L31 (-45, 103) -> (-45, 117)
  line L32 (45, 89) -> (46, 89)
  line L33 (46, 89) -> (46, 117)
  line L34 (46, 117) -> (45, 117)
  line L35 (45, 117) -> (45, 89)
  line L36 (45, 89) -> (44, 89)
  line L37 (44, 89) -> (44, 117)
  line L38 (44, 117) -> (45, 117)
  line L39 (45, 117) -> (45, 89)
  line L40 (15, 89) -> (16, 89)
  line L41 (16, 89) -> (16, 89)
  line L42 (16, 89) -> (15, 89)
  line L43 (15, 89) -> (15, 89)
  line L44 (16, 89) -> (14, 89)
  line L45 (14, 89) -> (14, 117)
  line L46 (14, 117) -> (16, 117)
  line L47 (16, 117) -> (16, 89)
  line L48 (-15, 89) -> (-14, 89)
  line L49 (-14, 89) -> (-14, 89)
  line L50 (-14, 89) -> (-15, 89)
  line L51 (-15, 89) -> (-15, 89)
  line L52 (-14, 89) -> (-16, 89)
  line L53 (-16, 89) -> (-16, 117)
  line L54 (-16, 117) -> (-14, 117)
  line L55 (-14, 117) -> (-14, 89)
  line L56 (-45, 89) -> (-44, 89)
  line L57 (-44, 89) -> (-44, 89)
  line L58 (-44, 89) -> (-45, 89)
  line L59 (-45, 89) -> (-45, 89)
  line L60 (-44, 89) -> (-46, 89)
  line L61 (-46, 89) -> (-46, 117)
  line L62 (-46, 117) -> (-44, 117)
  line L63 (-44, 117) -> (-44, 89)
  dimension "d157" = 1
  dimension "d158" = 2
  dimension "d159" = 2
  constraint coincident A9.centre L18.start
  constraint coincident A3.centre L18.end
  constraint coincident A5.centre L19.end
  constraint coincident A7.centre L20.end
  constraint coincident A1.centre L21.end
  constraint midpoint L19 L24.start
  constraint coincident L14 L24.end
  constraint perpendicular L14 L24
  constraint coincident L10 L25.end
  constraint perpendicular L10 L25
  constraint midpoint L20 L26.start
  constraint coincident L14 L26.end
  constraint perpendicular L14 L26
  constraint coincident L10 L27.end
  constraint perpendicular L10 L27
  constraint midpoint L21 L28.start
  constraint coincident L14 L28.end
  constraint perpendicular L14 L28
  constraint coincident L10 L29.end
  constraint perpendicular L10 L29
  constraint midpoint L22 L30.start
  constraint coincident L14 L30.end
  constraint perpendicular L14 L30
  constraint perpendicular L22 L31
  constraint horizontal L32
  constraint vertical L33
  constraint horizontal L34
  constraint vertical L35
  constraint horizontal L36
  constraint vertical L37
  constraint horizontal L38
  constraint vertical L39
  constraint coincident L10 L37.end
  constraint horizontal L40
  constraint horizontal L42
  constraint coincident L14 L40.end
  constraint horizontal L44
  constraint vertical L45
  constraint horizontal L46
  constraint vertical L47
  constraint horizontal L48
  constraint horizontal L50
  constraint coincident L14 L48.end
  constraint horizontal L52
  constraint vertical L53
  constraint horizontal L54
  constraint vertical L55
  constraint coincident L10 L53.end
  constraint horizontal L56
  constraint horizontal L58
  constraint coincident L14 L56.end
  constraint horizontal L60
  constraint vertical L61
  constraint horizontal L62
  constraint vertical L63
  measures "d157" distance of L24.end L32.end
  measures "d158" distance of L40.end L44.end
  measures "d159" distance of L56.end L60.end
move_body "Verschieben15" bodies 14 to x (1, 0, 0) y (0, 1, 0) z (0, 0, 1) at (0, -20, 0)
move_body "Verschieben16" bodies 14 to x (1, 0, 0) y (0, 1, 0) z (0, 0, 1) at (0, -80, 0)
sketch "Skizze27" plane through (75, 0, 0) normal (1, 0, 0) x (0, 1, 0)
  line L0 (46, 15) -> (49, 15)
  line L1 (49, 15) -> (49, 30)
  line L2 (49, 30) -> (-5, 30)
  line L3 (-5, 30) -> (-5, 15)
  line L4 (-5, 15) -> (28, 15)
  arc A0 (46, 15) -> (28, 15) centre (37, 15) ccw
  circle A1 centre (37, 15) radius 9.5
  circle A2 centre (37, 15) radius 11.5
  dimension "d160" = 19
  dimension "d161" = 23
  constraint concentric A0 A1
  constraint concentric A1 A2
  measures "d160" diameter of A1
  measures "d161" diameter of A2
extrude "Extrusion33" add sketch "Skizze27" along normal blind 25 separate body contours L0 L4 A1 A2 | L0 L4 A1 A2 makes body 15
sketch "Skizze28" plane through (100, 0, 0) normal (1, 0, 0) x (0, 1, 0)
  circle A0 centre (37, 15) radius 9.5
  circle A1 centre (37, 15) radius 11.5
  circle A2 centre (37, 15) radius 8
  dimension "d164" = 16
  constraint concentric A0 A2
  measures "d164" diameter of A2
extrude "Extrusion34" add sketch "Skizze28" against normal blind 18 contours A0 bodies 15
move_body "Verschieben17" bodies 2 3 8 5 9 to x (1, 0, 0) y (0, 1, 0) z (0, 0, 1) at (0, 50, 0)
move_body "Verschieben18" bodies 11 to x (1, 0, 0) y (0, 1, 0) z (0, 0, 1) at (0, 110, -13)
copy_body "Körper kopieren/einfügen4" bodies 15 makes body 16
move_body "Verschieben19" bodies 16 to x (0, -1, 0) y (1, 0, 0) z (0, 0, 1) at (23, 67, 0)
copy_body "Körper kopieren/einfügen5" bodies 16 makes body 17
move_body "Verschieben20" bodies 17 to x (1, 0, 0) y (0, 1, 0) z (0, 0, 1) at (-30, 0, 0)
copy_body "Körper kopieren/einfügen6" bodies 16 17 makes body 18 makes body 19
move_body "Verschieben21" bodies 18 19 to x (1, 0, 0) y (0, 1, 0) z (0, 0, 1) at (-60, 0, 0)
copy_body "Körper kopieren/einfügen7" bodies 19 makes body 20
move_body "Verschieben22" bodies 20 to x (1, 0, 0) y (0, 1, 0) z (0, 0, 1) at (-29.9817, 0, -1.047)
move_body "Verschieben23" bodies 11 to x (1, 0, 0) y (0, 1, 0) z (0, 0, 1) at (0, 0, 50)
move_body "Verschieben24" bodies 2 3 8 5 9 11 to x (1, 0, 0) y (0, 1, 0) z (0, 0, 1) at (0, 0, 40)
move_body "Verschieben25" bodies 11 to x (1, 0, 0) y (0, 1, 0) z (0, 0, 1) at (0, 0, -20)
move_body "Verschieben26" bodies 12 to x (1, 0, 0) y (0, 1, 0) z (0, 0, 1) at (0, 0, -60)
move_body "Verschieben27" bodies 20 19 18 17 16 to x (1, 0, 0) y (0, 1, 0) z (0, 0, 1) at (0, -30, 0)
move_body "Verschieben28" bodies 15 to x (1, 0, 0) y (0, 1, 0) z (0, 0, 1) at (25, 0, 0)
move_body "Verschieben29" bodies 8 5 9 2 3 to x (1, 0, 0) y (0, 1, 0) z (0, 0, 1) at (0, 0, -10)
move_body "Verschieben30" bodies 11 to x (1, 0, 0) y (0, 1, 0) z (0, 0, 1) at (0, 0, -30)
move_body "Verschieben31" bodies 12 to x (1, 0, 0) y (0, 1, 0) z (0, 0, 1) at (0, 0, 40)
move_body "Verschieben32" bodies 5 3 8 17 14 16 9 15 20 18 11 12 2 19 to x (1, 0, 0) y (0, 1, 0) z (0, 0, 1) at (0, 0, 20)
